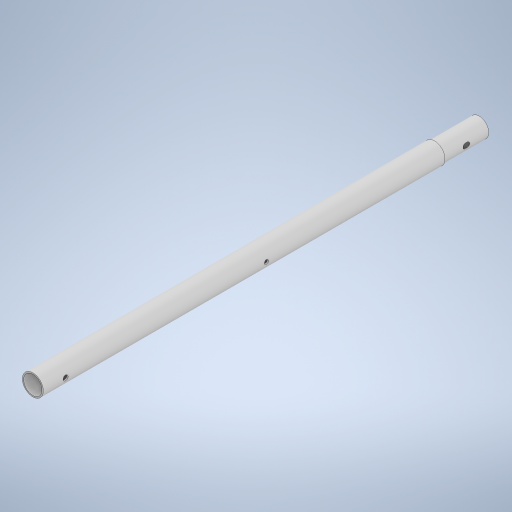
# Autodesk Inventor part: Część masztu 2 pod odciągi
Saved by Autodesk Inventor 2024 (Build 280153000, 153)
## iProperties
Created: 2024-11-10
Part Number: Część masztu 2 pod odciągi
Material: Generic
Document SubType Name: Modeling
Designer: Admin
Density: 1 g/cm^3
Appearance: Default
Author: Admin
Autodesk Inventor part; units mm, degrees
sketch "Sketch1" plane through (0, 0, 0) normal (0, 0, 1) x (1, 0, 0)
  circle A0 centre (0, 0) radius 23.5
  dimension "d0" = 47
  constraints: 1 centre point, 1 coincident
  measures "d0" diameter of A0
extrude "Extrusion1" add sketch "Sketch1" along normal blind 900
sketch "Sketch2" plane through (0, 0, 900) normal (0, 0, 1) x (1, 0, 0)
  circle A0 centre (0, 0) radius 20.5
  dimension "d3" = 41
  constraints: 1 centre point, 1 coincident
  measures "d3" diameter of A0
extrude "Extrusion2" cut sketch "Sketch2" against normal blind 900
sketch "Sketch3" plane through (0, 0, 0) normal (0, 0, -1) x (-1, 0, 0)
  circle A0 centre (0, 0) radius 21.5
  dimension "d6" = 43
  constraints: 1 centre point, 1 coincident
  measures "d6" diameter of A0
extrude "Extrusion3" add sketch "Sketch3" along normal blind 100
sketch "Sketch4" plane through (0, 0, -100) normal (0, 0, -1) x (-1, 0, 0)
  circle A0 centre (0, 0) radius 20.5
  dimension "d9" = 41
  constraints: 1 centre point, 1 coincident
  measures "d9" diameter of A0
extrude "Extrusion4" cut sketch "Sketch4" against normal blind 100
ref_plane "Work Plane1" through (23.5, 0, 0) normal (1, 0, 0) x (0, 1, 0)
sketch "Sketch5" plane through (23.5, 0, 0) normal (1, 0, 0) x (0, 1, 0)
  arc A0 (5.5, -48) -> (-5.5, -48) centre (0, -48) ccw
  arc A1 (-5.5, -52) -> (5.5, -52) centre (0, -52) ccw
  line L0 (23.5, 0) -> (-23.5, 0) projected
  line L1 (5.5, -48) -> (5.5, -52)
  line L2 (-5.5, -52) -> (-5.5, -48)
  point P0 (0, 0)
  point P1 (-5.5, -50)
  point P2 (5.5, -50)
  dimension "d13" = 11
  dimension "d14" = 48
  dimension "d15" = 11
  dimension "d16" = 52
  dimension "d17" = 11
  constraints: 4 end point, 4 point on circle, 3 tangent, 2 centre point, 2 midpoint
  measures "d13" diameter of A0
  measures "d14" distance of point (0, 0) A0.centre
  measures "d15" diameter of A1
  measures "d16" distance from line of L0 A1.centre
  measures "d17" distance of point (-5.5, -50) point (5.5, -50)
extrude "Extrusion5" cut sketch "Sketch5" against normal blind 47
sketch "Sketch6" plane through (23.5, 0, 0) normal (1, 0, 0) x (0, 1, 0)
  circle A0 centre (0, 850) radius 5.5
  line L0 (23.5, 900) -> (-23.5, 900) projected
  point P0 (0, 0)
  dimension "d20" = 11
  dimension "d21" = 50
  constraints: 1 centre point
  measures "d20" diameter of A0
  measures "d21" distance from line of L0 A0.centre
hole "Hole1" at (23.5, 0, 850) direction (-1, 0, 0) diameter 11 depth 47
ref_plane "Work Plane2" through (23.25, 0, 0) normal (1, 0, 0) x (0, 1, 0)
ref_plane "Work Plane3" through (30, 0, 0) normal (1, 0, 0) x (0, 1, 0)
sketch "Sketch8" plane through (30, 0, 0) normal (1, 0, 0) x (0, 1, 0)
  circle A0 centre (0, 400) radius 4.5
  line L0 (-21.5, -100) -> (21.5, -100) projected
  point P0 (0, 0)
  dimension "d40" = 9
  dimension "d41" = 500
  constraints: 1 centre point
  measures "d40" diameter of A0
  measures "d41" distance from line of L0 A0.centre
hole "Hole3" at (30, 0, 400) direction (-1, 0, 0) diameter 9 depth 50
ref_plane "Work Plane4" through (-31.75, 0, 0) normal (1, 0, 0) x (0, 1, 0)
sketch "Sketch9" plane through (-31.75, 0, 0) normal (1, 0, 0) x (0, 1, 0)
  circle A0 centre (0, 400) radius 4.5
  line L0 (-21.5, -100) -> (21.5, -100) projected
  point P0 (0, 0)
  dimension "d50" = 9
  dimension "d51" = 500
  constraints: 1 centre point
  measures "d50" diameter of A0
  measures "d51" distance from line of L0 A0.centre
hole "Hole4" at (-31.75, 0, 400) direction (1, 0, 0) diameter 9 depth 50
body "Solid1"
